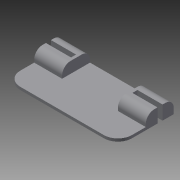
# Autodesk Inventor part: number holder
Saved by Autodesk Inventor 2015 (Build 190159000, 159)
## iProperties
Created: 2015-06-16
Part Number: number holder
Material: Generic
Document SubType Name: Modeling
Designer: Jason
Density: 1 g/cm^3
Appearance: Default
Author: Jason
Autodesk Inventor part; units mm, degrees
ref_plane "YZ Plane" through (0, 0, 0) normal (1, 0, 0) x (0, 1, 0)
ref_plane "XZ Plane" through (0, 0, 0) normal (0, 1, 0) x (-1, 0, 0)
ref_plane "XY Plane" through (0, 0, 0) normal (0, 0, 1) x (1, 0, 0)
sketch "Sketch1" plane through (0, 0, 0) normal (0, 0, 1) x (1, 0, 0)
  line L0 (2, 14) -> (42, 14)
  line L1 (42, 14) -> (42, -6)
  line L2 (42, -6) -> (2, -6)
  line L3 (2, -6) -> (2, 14)
  point P0 (0, 0)
  dimension "d0" = 40
  dimension "d1" = 20
  constraints: 8 end point, 2 parallel, 1 horizontal, 1 perpendicular
  measures "d0" distance of L1.end L2.end
  measures "d1" distance of L0.end L1.end
extrude "Extrusion1" add sketch "Sketch1" along normal blind 1
sketch "Sketch2" plane through (0, 0, 1) normal (0, 0, 1) x (1, 0, 0)
  line L0 (2, 14) -> (2, -6) projected
  line L1 (2, 14) -> (12, 14)
  line L2 (12, 14) -> (12, 4)
  line L3 (12, 4) -> (2, 4)
  line L4 (2, 4) -> (2, 14)
  line L5 (42, 14) -> (2, 14) projected
  line L6 (42, -6) -> (42, 14) projected
  line L7 (42, 14) -> (32, 14)
  line L8 (32, 14) -> (32, 4)
  line L9 (32, 4) -> (42, 4)
  line L10 (42, 4) -> (42, 14)
  point P0 (0, 0)
  dimension "d4" = 10
  dimension "d5" = 0
  dimension "d6" = 10
  dimension "d7" = 10
  dimension "d8" = 10
  dimension "d9" = 0
  constraints: 16 end point, 4 parallel, 2 horizontal, 2 perpendicular, 2 point on line
  measures "d4" distance of L1.end L2.end
  measures "d5" distance between parallel lines of L5 L1
  measures "d6" distance of L1.start L1.end
  measures "d7" distance of L9.end L8.end
  measures "d8" distance of L8.end L7.end
  measures "d9" distance between parallel lines of L5 L7
extrude "Extrusion2" add sketch "Sketch2" along normal blind 4
sketch "Sketch3" plane through (0, 0, 5) normal (0, 0, 1) x (1, 0, 0)
  line L0 (2, 10) -> (11, 10)
  line L1 (11, 10) -> (11, 8.2)
  line L2 (11, 8.2) -> (2, 8.2)
  line L3 (2, 8.2) -> (2, 10)
  line L4 (42, 10) -> (33, 10)
  line L5 (33, 10) -> (33, 8.2)
  line L6 (33, 8.2) -> (42, 8.2)
  line L7 (42, 8.2) -> (42, 10)
  line L8 (32, 14) -> (12, 14) projected
  line L9 (32, 14) -> (12, 14) projected
  line L10 (32, 14) -> (32, 4) projected
  line L11 (12, 4) -> (12, 14) projected
  point P0 (0, 0)
  point P1 (2, 9)
  point P2 (42, 9)
  dimension "d12" = 9
  dimension "d13" = 1.8
  dimension "d14" = 9
  dimension "d15" = 1.8
  dimension "d16" = 4
  dimension "d17" = 4
  dimension "d22" = 1
  dimension "d23" = 1
  constraints: 16 end point, 4 parallel, 2 horizontal, 2 perpendicular, 2 other
  measures "d12" distance of L1.end L2.end
  measures "d13" distance of L0.end L1.end
  measures "d14" distance of L6.end L5.end
  measures "d15" distance of L5.end L4.end
  measures "d22" distance between parallel lines of L10 L5
  measures "d23" distance between parallel lines of L1 L11
extrude "Extrusion3" cut sketch "Sketch3" against normal through all
fillet "Fillet1" radius 3 4 edges at (37, 14, 5) (37, 4, 5) (7, 4, 5) (7, 14, 5)
fillet "Fillet2" radius 5 2 edges at (2, -6, 0.5) (42, -6, 0.5)
body "Solid1"
